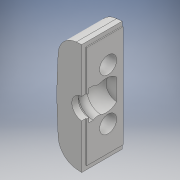
# Autodesk Inventor part: Part1
Saved by Autodesk Inventor 2017 (Build 210142000, 142)
## iProperties
Created: 2019-06-26
Part Number: Part1
Material: Generic
Document SubType Name: Modeling
Designer: Ole Simmering
Density: 1 g/cm^3
Appearance: Default
Author: Ole Simmering
Autodesk Inventor part; units mm, degrees
ref_plane "YZ Plane" through (0, 0, 0) normal (1, 0, 0) x (0, 1, 0)
ref_plane "XZ Plane" through (0, 0, 0) normal (0, 1, 0) x (-1, 0, 0)
ref_plane "XY Plane" through (0, 0, 0) normal (0, 0, 1) x (1, 0, 0)
sketch "Sketch1" plane through (0, 0, 0) normal (0, 1, 0) x (-1, 0, 0)
  line L0 (0, 0) -> (0, -26)
  line L1 (0, -26) -> (1.5, -25.8688)
  line L2 (-5, -13) -> (15, -13) construction
  line L3 (0, 0) -> (1.5, -0.1312)
  arc A0 (1.5, -25.8688) -> (5.6905, -21.6131) centre (1.0988, -21.2827) ccw
  arc A1 (5.6905, -4.3869) -> (1.5, -0.1312) centre (1.0988, -4.7173) ccw
  arc A2 (5.6905, -21.6131) -> (6, -13) centre (-114, -13) ccw
  arc A3 (6, -13) -> (5.6905, -4.3869) centre (-114, -13) ccw
  dimension "d0" = 26
  dimension "d5" = 85
  dimension "d6" = 1.5
  dimension "d7" = 6
  dimension "d8" = 120
  constraints: 8 end point, 8 point on circle, 4 centre point, 4 symmetric about line, 2 tangent, 1 horizontal, 1 point on line, 1 vertical, 1 other
  measures "d0" distance of L0.start L0.end
  measures "d5" angle of L1 L0
  measures "d6" distance from line of L1.end L0
  measures "d7" distance from line of A2.end L0
  measures "d8" radius of A2
extrude "Extrusion1" add sketch "Sketch1" along normal blind 9.5
ref_plane "Work Plane1" through (-6, 0, 0) normal (1, 0, 0) x (0, 0, -1)
sketch "Sketch2" plane through (-6, 0, 0) normal (1, 0, 0) x (0, 0, -1)
  line L0 (0, 9.5) -> (26, 9.5) construction
  line L1 (7, 9.5) -> (7, 0) construction
  line L2 (0, 0) -> (26, 0) construction
  line L3 (0, 0) -> (0, 9.5) construction
  line L4 (0, 6) -> (26, 6) construction
  line L5 (19, 9.5) -> (19, 0) construction
  line L6 (0, 0) -> (26, 0) construction
  line L7 (26, 0) -> (26, 9.5) construction
  line L8 (0, 9.5) -> (26, 9.5) construction
  line L9 (0, 0) -> (0, 9.5) construction
  line L10 (13, 10.3303) -> (13, -1) construction
  point P0 (7, 6)
  point P1 (19, 6)
  dimension "d11" = 6
  dimension "d12" = 7
  constraints: 14 end point, 6 point on line, 1 horizontal, 1 vertical
  measures "d11" distance between parallel lines of L2 L4
  measures "d12" distance between parallel lines of L3 L1
hole "Hole1" at (-6, 6, -7) at (-6, 6, -19) direction (1, 0, 0) diameter 2 end through all countersink diameter 4 countersink angle 90
sketch "Sketch3" plane through (0, 0, 0) normal (1, 0, 0) x (0, 0, -1)
  circle A0 centre (7, 6) radius 1 projected
  circle A1 centre (19, 6) radius 1 projected
  point P0 (0, 0)
  constraints: 2 coincident
hole "Hole2" at (0, 6, -7) at (0, 6, -19) direction (-1, 0, 0) diameter 4 depth 3 tip angle 118
sketch "Sketch4" plane through (0, 0, 0) normal (1, 0, 0) x (0, 0, -1)
  circle A0 centre (7, 6) radius 2 projected
  circle A1 centre (19, 6) radius 2 projected
  line L0 (0, 0) -> (26, 0) projected
  line L1 (26, 0) -> (26, 9.5) projected
  line L2 (0, 9.5) -> (26, 9.5) construction
  line L3 (0, 0) -> (0, 9.5) projected
  line L4 (1, 9.5) -> (1, 1)
  line L5 (1, 1) -> (25, 1)
  line L6 (25, 1) -> (25, 9.5)
  line L7 (0, 0) -> (0, 9.5) projected
  line L8 (0, 9.5) -> (1, 9.5)
  line L9 (26, 0) -> (26, 9.5) projected
  line L10 (25, 9.5) -> (26, 9.5)
  dimension "d28" = 1
  dimension "d29" = 1
  dimension "d30" = 1
  constraints: 10 end point, 2 perpendicular, 2 point on line, 1 horizontal, 1 parallel, 1 vertical
  measures "d28" distance between parallel lines of L3 L4
  measures "d29" distance between parallel lines of L0 L5
  measures "d30" distance between parallel lines of L1 L6
extrude "Extrusion2" cut sketch "Sketch4" against normal blind 0.2 contours L3 L8 L4 L5 L6 L10 L1 L0
sketch "Sketch5" plane through (0, 0, 0) normal (0, -1, 0) x (1, 0, 0)
  line L0 (0, -1) -> (0, -25) projected
  circle A0 centre (0, -13) radius 2.5
  point P0 (0, 0)
  dimension "d33" = 5
  constraints: 1 centre point, 1 midpoint
  measures "d33" diameter of A0
extrude "Extrusion3" cut sketch "Sketch5" against normal blind 7
sketch "Sketch6" plane through (0, 1, -25) normal (1, 0, 0) x (0, 0, -1)
  line L0 (-14.5, 6) -> (-9.5, 6) construction
  line L1 (-14.5, 0) -> (-14.5, 6) construction
  arc A0 (-14.5, 2.101) -> (-12, 1.0505) centre (-12, 4.5505) ccw construction
  line L2 (-14.5, 7) -> (-12, 7) construction
  line L3 (-3.3869, 8.5) -> (-20.6131, 8.5) construction
  line L4 (-12, 8.5) -> (-12, -2) construction
  arc A1 (-14.5, 7) -> (-14.5, 2.101) centre (-12, 4.5505) ccw construction
  arc A2 (-9.5, 7) -> (-14.5, 7) centre (-12, 4.5505) ccw construction
  line L5 (-12, 7) -> (-9.5, 7)
  arc A3 (-12, 1.0505) -> (-9.5, 7) centre (-12, 4.5505) ccw
  line L6 (-12, 7) -> (-12, 1.0505)
  point P0 (-25, -1)
  dimension "d36" = 7
  dimension "d37" = 1.5
  dimension "d38" = 5
  constraints: 8 end point, 8 point on circle, 4 centre point, 4 point on line, 2 horizontal, 2 perpendicular, 1 midpoint, 1 symmetric about line
  measures "d36" diameter of A0
  measures "d37" distance between parallel lines of L3 L2
  measures "d38" distance of L2.start L5.end
revolve "Revolution1" cut sketch "Sketch6" angle 360 about axis through (0, 9.5, -13) along (0, -1, 0)
sketch "Sketch7" plane through (0, 1, -25) normal (1, 0, 0) x (0, 0, -1)
  line L0 (-12, 0.5) -> (-8.5, 0.5)
  line L1 (-8.5, 0.5) -> (-8.5, 1.5)
  line L2 (-8.5, 1.5) -> (-12, 1.5)
  line L3 (-12, 1.5) -> (-12, 0.5)
  line L4 (-9.5, 7) -> (-14.5, 7) construction
  line L5 (-12, 7) -> (-12, -2.0028) construction
  line L6 (-9.508, -1) -> (-14.492, -1) construction
  point P0 (-25, -1)
  dimension "d41" = 3.5
  dimension "d42" = 1
  dimension "d43" = 1.5
  constraints: 10 end point, 2 parallel, 1 horizontal, 1 midpoint, 1 perpendicular, 1 vertical
  measures "d41" distance of L0.start L0.end
  measures "d42" distance of L0.end L1.end
  measures "d43" distance between parallel lines of L6 L0
revolve "Revolution2" cut sketch "Sketch7" angle 360 about axis through (0, 2.5, -13) along (0, -1, 0)
fillet "Fillet1" radius 2 2 edges at (-2.5, 3.101, -13) (-2.5, 2.5, -13)
equation "\"d30\" = d28"
body "Solid1"
